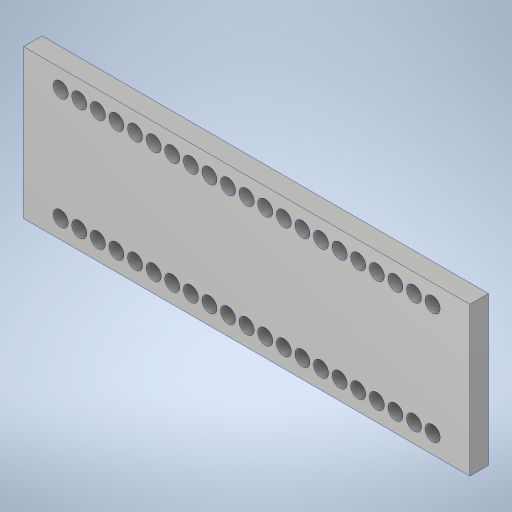
# Autodesk Inventor part: Gp1-001
Saved by Autodesk Inventor 2023.4 (Build 274418000, 418)
## iProperties
Created: 2025-01-05
Part Number: Gp1-001
Material: Aluminum 6061
Document SubType Name: Modeling
Designer: mavericks
Density: 2.7 g/cm^3
Appearance: Aluminum - Flat
Author: mavericks
Autodesk Inventor part; units mm, degrees
ref_plane "YZ Plane" through (0, 0, 0) normal (1, 0, 0) x (0, 1, 0)
ref_plane "XZ Plane" through (0, 0, 0) normal (0, 1, 0) x (-1, 0, 0)
ref_plane "XY Plane" through (0, 0, 0) normal (0, 0, 1) x (1, 0, 0)
sketch "Sketch1" plane through (0, 0, 0) normal (0, 0, 1) x (1, 0, 0)
  line L0 (-76.2, 25.4) -> (76.2, 25.4)
  line L1 (76.2, 25.4) -> (76.2, -25.4)
  line L2 (76.2, -25.4) -> (-76.2, -25.4)
  line L3 (-76.2, -25.4) -> (-76.2, 25.4)
  line L4 (-76.2, 25.4) -> (76.2, -25.4) construction
  line L5 (76.2, 25.4) -> (-76.2, -25.4) construction
  point P0 (0, 0)
  dimension "d0" = 152.4
  dimension "d1" = 50.8
  constraints: 12 end point, 2 midpoint, 2 parallel, 1 horizontal, 1 perpendicular
  measures "d0" distance of L1.end L2.end
  measures "d1" distance of L0.end L1.end
extrude "Extrusion1" add sketch "Sketch1" along normal blind 6.35
sketch "Sketch2" plane through (0, 0, 6.35) normal (0, 0, 1) x (1, 0, 0)
  line L0 (-76.2, 25.4) -> (-76.2, -25.4) construction
  line L1 (76.2, 25.4) -> (-76.2, 25.4) construction
  line L2 (-43.7106, 0) -> (44.45, 0) construction
  line L3 (-76.2, -25.4) -> (76.2, -25.4) construction
  point P0 (0, 0)
  point P1 (-63.5, 19.05)
  point P2 (-57.15, 19.05)
  point P3 (-50.8, 19.05)
  point P4 (-44.45, 19.05)
  point P5 (-38.1, 19.05)
  point P6 (-31.75, 19.05)
  point P7 (-25.4, 19.05)
  point P8 (-19.05, 19.05)
  point P9 (-12.7, 19.05)
  point P10 (-6.35, 19.05)
  point P11 (0, 19.05)
  point P12 (6.35, 19.05)
  point P13 (12.7, 19.05)
  point P14 (19.05, 19.05)
  point P15 (25.4, 19.05)
  point P16 (31.75, 19.05)
  point P17 (38.1, 19.05)
  point P18 (44.45, 19.05)
  point P19 (50.8, 19.05)
  point P20 (57.15, 19.05)
  point P21 (63.5, 19.05)
  point P22 (-63.5, -19.05)
  point P23 (-57.15, -19.05)
  point P24 (-50.8, -19.05)
  point P25 (-44.45, -19.05)
  point P26 (-38.1, -19.05)
  point P27 (-31.75, -19.05)
  point P28 (-25.4, -19.05)
  point P29 (-19.05, -19.05)
  point P30 (-12.7, -19.05)
  point P31 (-6.35, -19.05)
  point P32 (0, -19.05)
  point P33 (6.35, -19.05)
  point P34 (12.7, -19.05)
  point P35 (19.05, -19.05)
  point P36 (25.4, -19.05)
  point P37 (31.75, -19.05)
  point P38 (38.1, -19.05)
  point P39 (44.45, -19.05)
  point P40 (50.8, -19.05)
  point P41 (57.15, -19.05)
  point P42 (63.5, -19.05)
  dimension "d4" = 12.7
  dimension "d5" = 6.35
  dimension "d8" = 6.35
  dimension "d13" = 6.35
  constraints: 21 symmetric about line, 2 end point, 2 horizontal, 20 other
  measures "d4" distance from line of point (-63.5, 19.05) L0
  measures "d5" distance from line of point (-63.5, 19.05) L1
  measures "d8" distance of point (-63.5, 19.05) point (-57.15, 19.05)
  measures "d13" distance from line of L3 point (-63.5, -19.05)
hole "Hole1" at (-63.5, 19.05, 6.35) at (-57.15, 19.05, 6.35) at (-50.8, 19.05, 6.35) at (-44.45, 19.05, 6.35) at (-38.1, 19.05, 6.35) at (-31.75, 19.05, 6.35) at (-25.4, 19.05, 6.35) at (-19.05, 19.05, 6.35) at (-12.7, 19.05, 6.35) at (-6.35, 19.05, 6.35) at (0, 19.05, 6.35) at (6.35, 19.05, 6.35) at (12.7, 19.05, 6.35) at (19.05, 19.05, 6.35) at (25.4, 19.05, 6.35) at (31.75, 19.05, 6.35) at (38.1, 19.05, 6.35) at (44.45, 19.05, 6.35) at (50.8, 19.05, 6.35) at (57.15, 19.05, 6.35) at (63.5, 19.05, 6.35) at (63.5, -19.05, 6.35) at (57.15, -19.05, 6.35) at (50.8, -19.05, 6.35) at (44.45, -19.05, 6.35) at (38.1, -19.05, 6.35) at (31.75, -19.05, 6.35) at (25.4, -19.05, 6.35) at (19.05, -19.05, 6.35) at (12.7, -19.05, 6.35) at (6.35, -19.05, 6.35) at (0, -19.05, 6.35) at (-6.35, -19.05, 6.35) at (-12.7, -19.05, 6.35) at (-19.05, -19.05, 6.35) at (-25.4, -19.05, 6.35) at (-31.75, -19.05, 6.35) at (-38.1, -19.05, 6.35) at (-44.45, -19.05, 6.35) at (-50.8, -19.05, 6.35) at (-57.15, -19.05, 6.35) at (-63.5, -19.05, 6.35) direction (0, 0, -1) diameter 5.1054 end through all clearance for "Flat Head Machine Screw (82)" size "#10" standard "Ansi Unified Screw Threads"
body "Solid1"
